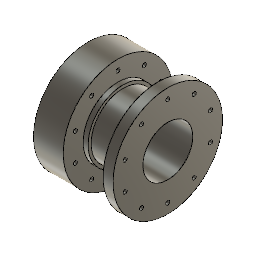
primary_turbine_bushing_Eng_model (Autodesk Fusion 360 design; units mm, degrees)
Autodesk Fusion 360 part; units mm, degrees
sketch "Sketch1" plane through (0, 0, 0) normal (0, 1, 0) x (1, 0, 0)
  line L0 (0, 0) -> (131.5429, 0) construction
  line L1 (80, 0) -> (80, -25) construction
  line L2 (80, -25) -> (20, -25)
  line L3 (80, -25) -> (80, -55)
  line L4 (80, -55) -> (70, -55)
  line L5 (70, -55) -> (70, -35)
  line L6 (70, -35) -> (65, -35)
  line L7 (65, -35) -> (65, -32)
  line L8 (65, -32) -> (35, -32)
  line L9 (35, -32) -> (35, -35)
  line L10 (35, -35) -> (30, -35)
  line L11 (30, -35) -> (30, -55)
  line L12 (30, -55) -> (0, -55)
  line L13 (20, -25) -> (20, -35)
  line L14 (0, -35) -> (20, -35)
  line L15 (0, -50) -> (20, -50)
  line L16 (20, -50) -> (20, -40)
  line L17 (20, -40) -> (0, -40)
  line L18 (0, -55) -> (0, -50)
  line L19 (0, -40) -> (0, -35)
  dimension "d1" = 25
  dimension "d2" = 80
  dimension "d3" = 60
  dimension "d4" = 55
  dimension "d5" = 10
  dimension "d6" = 20
  dimension "d7" = 5
  dimension "d8" = 3
  dimension "d9" = 30
  dimension "d10" = 3
  dimension "d11" = 5
  dimension "d12" = 55
  dimension "d13" = 30
  dimension "d14" = 20
  dimension "d15" = 35
  dimension "d16" = 10
  dimension "d17" = 5
  dimension "d18" = 5
  dimension "d19" = 20
  constraint coincident L0.start origin
  constraint horizontal L0
  constraint coincident L0 L1.start
  constraint perpendicular L0 L1
  constraint perpendicular L1 L2
  constraint perpendicular L2 L3
  constraint perpendicular L3 L4
  constraint perpendicular L4 L5
  constraint perpendicular L5 L6
  constraint perpendicular L6 L7
  constraint perpendicular L7 L8
  constraint perpendicular L8 L9
  constraint perpendicular L9 L10
  constraint perpendicular L10 L11
  constraint perpendicular L11 L12
  constraint perpendicular L12 L18
  constraint perpendicular L2 L13
  constraint perpendicular L15 L18
  constraint perpendicular L15 L16
  constraint coincident L17.end L18
  constraint perpendicular L17 L18
  constraint collinear L18 L19
  measures "d1" distance of L1.start L1.end
  measures "d2" distance of L0.start L1
  measures "d3" distance of L1.end L2.end
  measures "d4" distance of L1.start L3.end
  measures "d5" distance of L3.end L4.end
  measures "d6" distance of L4.end L5.end
  measures "d7" distance of L5.end L6.end
  measures "d8" distance of L6.end L7.end
  measures "d9" distance of L7.end L8.end
  measures "d10" distance of L8.end L9.end
  measures "d11" distance of L9.end L10.end
  measures "d12" distance of L0 L11.end
  measures "d13" distance of L11.end L12.end
  measures "d14" distance of L12.end L14.start
  measures "d15" distance of L0 L13.end
  measures "d16" distance of L15.end L16.end
  measures "d17" distance of L14 L17
  measures "d18" distance of L12 L15
  measures "d19" distance of L16 L18
revolve "Revolve1" add sketch "Sketch1" angle 360 about axis through (0, 0, 0) along (1, 0, 0)
sketch "Sketch2" plane through (80, 0, 0) normal (1, 0, 0) x (0, 1, 0)
  circle A0 centre (0, 0) radius 25
  circle A1 centre (0, 0) radius 55
  circle A2 centre (0, 45) radius 2
  line L0 (0, 55) -> (0, 62.9833) construction
  dimension "d21" = 4
  dimension "d22" = 45
  constraint coincident A1 L0.start
  measures "d21" diameter of A2
  measures "d22" distance of A0.centre A2.centre
extrude "Extrude1" cut sketch "Sketch2" along normal mid plane 170 contours A2
pattern_circular "C-Pattern1" count 10 over 360 about axis through (1.75, 0, 0) along (1, 0, 0) of "Extrude1"
